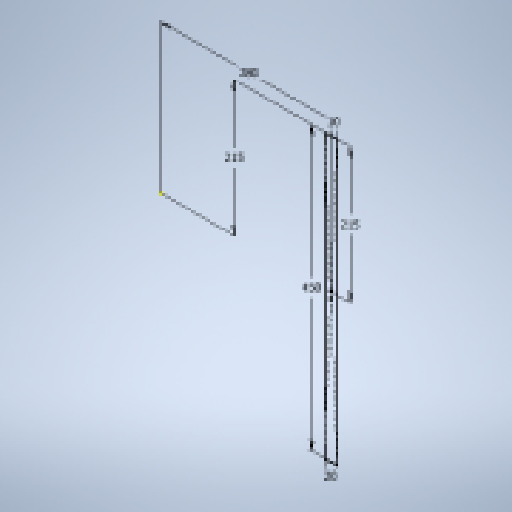
# Autodesk Inventor part: DOF1
Saved by Autodesk Inventor 2024 (Build 280153000, 153)
## iProperties
Created: 2024-10-15
Part Number: DOF1
Material: 一般
Document SubType Name: Modeling
Designer: jerry
Density: 1 g/cm^3
Appearance: 預設
Author: jerry
Autodesk Inventor part; units mm, degrees
ref_plane "YZ Plane" through (0, 0, 0) normal (1, 0, 0) x (0, 1, 0)
ref_plane "XZ Plane" through (0, 0, 0) normal (0, 1, 0) x (-1, 0, 0)
ref_plane "XY Plane" through (0, 0, 0) normal (0, 0, 1) x (1, 0, 0)
sketch "草圖1" plane through (0, 0, 0) normal (0, 0, 1) x (1, 0, 0)
  line L0 (280, 215) -> (260, 215)
  line L1 (260, 215) -> (260, -235)
  line L2 (260, -235) -> (280, -235)
  line L3 (280, -235) -> (280, 215)
  line L4 (280, 215) -> (260, -235) construction
  line L5 (260, 215) -> (280, -235) construction
  circle A0 centre (270, 190) radius 3
  circle A1 centre (270, -210) radius 3
  circle A2 centre (270, 12.5) radius 3
  circle A3 centre (270, -32.5) radius 3
  point P0 (0, 0)
  point P1 (270, -10)
  dimension "d3" = 20
  dimension "d4" = 450
  dimension "d5" = 280
  dimension "d6" = 215
  dimension "d8" = 225
  dimension "d11" = 6
  dimension "d12" = 6
  dimension "d14" = 6
  dimension "d15" = 6
  dimension "d16" = 10
  dimension "d17" = 25
  dimension "d18" = 10
  dimension "d19" = 202.5
  dimension "d20" = 10
  dimension "d21" = 10
  dimension "d22" = 247.5
  dimension "d23" = 10
  dimension "d24" = 425
  constraints: 12 end point, 4 centre point, 2 parallel, 1 horizontal, 1 perpendicular
  measures "d3" distance of L2.end L1.end
  measures "d4" distance of L1.end L0.end
  measures "d5" distance from line of point (0, 0) L3
  measures "d6" distance from line of point (0, 0) L0
  measures "d8" distance from line of point (270, -10) L0
  measures "d11" diameter of A0
  measures "d12" diameter of A1
  measures "d14" diameter of A2
  measures "d15" diameter of A3
  measures "d16" distance from line of A0.centre L3
  measures "d17" distance from line of A0.centre L0
  measures "d18" distance from line of A2.centre L3
  measures "d19" distance from line of A2.centre L0
  measures "d20" distance from line of point (270, -10) L3
  measures "d21" distance from line of A3.centre L3
  measures "d22" distance from line of A3.centre L0
  measures "d23" distance from line of A1.centre L3
  measures "d24" distance from line of A1.centre L0
extrude "擠出1" add sketch "草圖1" along normal blind 20
